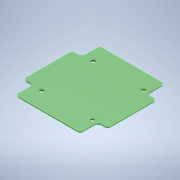
# Autodesk Inventor part: pcbIO
Saved by Autodesk Inventor 2021 (Build 250183000, 183)
## iProperties
Created: 2023-08-06
Part Number: pcbIO
Material: Generic
Document SubType Name: Modeling
Designer: michal
Density: 1 g/cm^3
Appearance: Smooth - Dark Forest Green
Author: michal
Autodesk Inventor part; units mm, degrees
ref_plane "YZ Plane" through (0, 0, 0) normal (1, 0, 0) x (0, 1, 0)
ref_plane "XZ Plane" through (0, 0, 0) normal (0, 1, 0) x (-1, 0, 0)
ref_plane "XY Plane" through (0, 0, 0) normal (0, 0, 1) x (1, 0, 0)
sketch "Sketch1" plane through (0, 0, 0) normal (0, 1, 0) x (-1, 0, 0)
  line L0 (-47.5, 47.5) -> (47.5, 47.5)
  line L1 (47.5, 47.5) -> (47.5, -47.5)
  line L2 (47.5, -47.5) -> (-47.5, -47.5)
  line L3 (-47.5, -47.5) -> (-47.5, 47.5)
  line L4 (-47.5, 47.5) -> (47.5, -47.5) construction
  line L5 (47.5, 47.5) -> (-47.5, -47.5) construction
  point P0 (0, 0)
  dimension "d0" = 95
  dimension "d1" = 95
  constraints: 12 end point, 2 midpoint, 2 parallel, 1 horizontal, 1 perpendicular
  measures "d0" distance of L1.end L2.end
  measures "d1" distance of L0.end L1.end
extrude "Extrusion1" add sketch "Sketch1" along normal blind 1.6
sketch "Sketch4" plane through (0, 1.6, 0) normal (0, 1, 0) x (1, 0, 0)
  line L0 (-47.5, 47.5) -> (-47.5, -47.5) projected
  line L1 (-47.5, -47.5) -> (-36.5, -47.5)
  line L2 (-36.5, -47.5) -> (-36.5, -27.5)
  line L3 (-36.5, -27.5) -> (-47.5, -27.5)
  line L4 (-47.5, -27.5) -> (-47.5, -47.5)
  line L5 (-47.5, -47.5) -> (47.5, -47.5) projected
  line L6 (47.5, -47.5) -> (36.5, -47.5)
  line L7 (36.5, -47.5) -> (36.5, -27.5)
  line L8 (36.5, -27.5) -> (47.5, -27.5)
  line L9 (47.5, -27.5) -> (47.5, -47.5)
  line L10 (-47.5, 47.5) -> (-36.5, 47.5)
  line L11 (-36.5, 47.5) -> (-36.5, 27.5)
  line L12 (-36.5, 27.5) -> (-47.5, 27.5)
  line L13 (-47.5, 27.5) -> (-47.5, 47.5)
  line L14 (47.5, 47.5) -> (-47.5, 47.5) projected
  line L15 (47.5, 47.5) -> (36.5, 47.5)
  line L16 (36.5, 47.5) -> (36.5, 27.5)
  line L17 (36.5, 27.5) -> (47.5, 27.5)
  line L18 (47.5, 27.5) -> (47.5, 47.5)
  point P0 (0, 0)
  point P1 (-47.5, -27.5)
  point P2 (-47.5, 27.5)
  dimension "d18" = 11
  dimension "d19" = 20
  dimension "d21" = 20
  dimension "d22" = 11
  dimension "d23" = 11
  dimension "d24" = 20
  dimension "d25" = 11
  dimension "d26" = 20
  constraints: 32 end point, 8 parallel, 4 horizontal, 4 perpendicular
  measures "d18" distance of L3.end L2.end
  measures "d19" distance of L2.end L1.end
  measures "d21" distance of L6.end L7.end
  measures "d22" distance of L16.end L17.end
  measures "d23" distance of L11.end L12.end
  measures "d24" distance of L15.end L16.end
  measures "d25" distance of L7.end L8.end
  measures "d26" distance of L10.end L11.end
extrude "Extrusion2" cut sketch "Sketch4" against normal blind 1.6
fillet "Fillet1" radius 4 4 edges at (36.5, 0.8, -27.5) (36.5, 0.8, 27.5) (-36.5, 0.8, 27.5) (-36.5, 0.8, -27.5)
fillet "Fillet2" radius 3 8 edges at (36.5, 0.8, 47.5) (-36.5, 0.8, 47.5) (-36.5, 0.8, -47.5) (36.5, 0.8, -47.5) (-47.5, 0.8, -27.5) (47.5, 0.8, -27.5) (47.5, 0.8, 27.5) (-47.5, 0.8, 27.5)
sketch "Sketch6" plane through (0, 1.6, 0) normal (0, 1, 0) x (1, 0, 0)
  line L0 (31.5, 29) -> (-25.5, 29) construction
  line L1 (-25.5, 29) -> (-25.5, -29) construction
  line L2 (-25.5, -29) -> (31.5, -29) construction
  line L3 (31.5, -29) -> (31.5, 29) construction
  line L4 (31.5, 29) -> (-25.5, -29) construction
  line L5 (-25.5, 29) -> (31.5, -29) construction
  line L6 (-66.5, 0) -> (66.5, 0) construction
  line L7 (0, 66.5) -> (0, -66.5) construction
  point P0 (3, 0)
  dimension "d31" = 57
  dimension "d32" = 58
  dimension "d41" = 3
  constraints: 13 end point, 3 coincident, 2 parallel, 1 horizontal, 1 midpoint, 1 perpendicular, 1 point on line
  measures "d31" distance of L0.start L0.end
  measures "d32" distance of L0.end L1.end
  measures "d41" distance from line of point (3, 0) L7
hole "Hole2" at (-25.5, 1.6, 29) at (-25.5, 1.6, -29) at (31.5, 1.6, -29) at (31.5, 1.6, 29) direction (0, -1, 0) diameter 4.2 end through all
equation "\"d19\" = d21"
equation "\"d22\" = d18"
equation "\"d23\" = d18"
equation "\"d24\" = d19"
equation "\"d25\" = d18"
equation "\"d26\" = d21"
body "Solid1"
